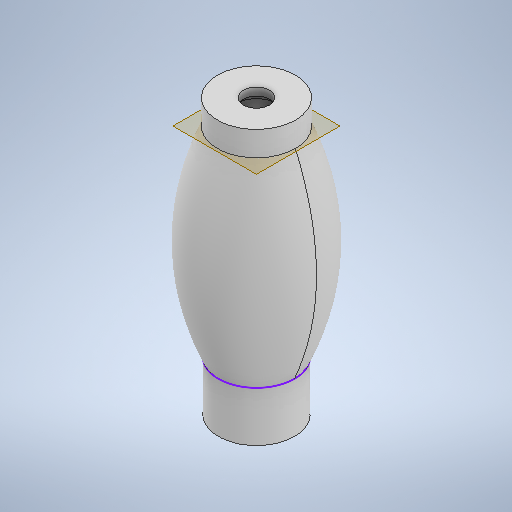
# Autodesk Inventor part: Pressure tank, 3d print. rev 001 inventor file
Saved by Autodesk Inventor 2025.2 (Build 292293000, 293)
## iProperties
Created: 2025-03-20
Part Number: Pressure tank, 3d print. rev 001 inventor file
Material: Generic
Document SubType Name: Modeling
Designer: Tobias
Density: 1 g/cm^3
Appearance: Default
Author: Tobias
## iProperties of the stored document Pressure tank, 3d print. rev 001 inventor file_3DPrint.ipt
Created: 2025-03-20
Part Number: Pressure tank, 3d print. rev 001 inventor file_3DPrint
Material: Generic
Document SubType Name: Modeling
Designer: Tobias
Density: 1 g/cm^3
Appearance: Default
Author: Tobias
Autodesk Inventor part; units mm, degrees
ref_plane "YZ Plane" through (0, 0, 0) normal (1, 0, 0) x (0, 1, 0)
ref_plane "XZ Plane" through (0, 0, 0) normal (0, 1, 0) x (-1, 0, 0)
ref_plane "XY Plane" through (0, 0, 0) normal (0, 0, 1) x (1, 0, 0)
sketch "Sketch1" plane through (0, 0, 0) normal (0, 1, 0) x (-1, 0, 0)
  circle A0 centre (0, 0) radius 15
  circle A1 centre (0, 0) radius 19
  dimension "d0" = 30
  dimension "d1" = 38
  constraints: 2 centre point, 2 coincident
  measures "d0" diameter of A0
  measures "d1" diameter of A1
extrude "Extrusion1" add sketch "Sketch1" along normal blind 25 contours A0 | A1
sketch "Sketch2" plane through (0, 25, 0) normal (0, 1, 0) x (1, 0, 0)
  circle A0 centre (0, 0) radius 19
  constraints: 1 centre point, 1 coincident
ref_plane "Work Plane1" through (0, 75, 0) normal (0, 1, 0) x (1, 0, 0)
sketch "Sketch3" plane through (0, 75, 0) normal (0, 1, 0) x (1, 0, 0)
  circle A0 centre (0, 0) radius 30
  dimension "d5" = 60
  constraints: 1 centre point, 1 coincident
  measures "d5" diameter of A0
ref_plane "Work Plane2" through (0, 125, 0) normal (0, 1, 0) x (1, 0, 0)
sketch "Sketch4" plane through (0, 125, 0) normal (0, 1, 0) x (1, 0, 0)
  point P0 (0, 0)
sketch "Sketch5" plane through (0, 125, 0) normal (0, 1, 0) x (1, 0, 0)
  circle A0 centre (0, 0) radius 19.5
  dimension "d7" = 39
  constraints: 1 centre point, 1 coincident
  measures "d7" diameter of A0
loft "Loft1" add profiles "Sketch3", "Sketch5" section 1 edges at (19, 25, 0)
sketch "Sketch7" plane through (0, 0, 0) normal (0, -1, 0) x (1, 0, 0)
  point P0 (0, 0)
  point P1 (0, 0)
  constraints: 1 coincident
hole "Hole1" at (0, 0, 0) direction (0, 1, 0) diameter 19.842 end through all clearance for "Hex Head Bolt" size "3/4" standard "Ansi Unified Screw Threads"
sketch "Sketch8" plane through (0, 125, 0) normal (0, 1, 0) x (1, 0, 0)
  circle A0 centre (0, 0) radius 19.5
  constraints: 1 centre point, 1 coincident
extrude "Extrusion2" add sketch "Sketch8" along normal blind 12.3
sketch "Sketch9" plane through (0, 137.3, 0) normal (0, 1, 0) x (1, 0, 0)
  point P0 (0, 0)
  point P1 (0, 0)
  constraints: 1 coincident
hole "Hole2" at (0, 137.3, 0) direction (0, -1, 0) diameter 13 depth 42.05 tip angle 118
sketch "Sketch10" plane through (0, 25, 0) normal (0, 1, 0) x (1, 0, 0)
  circle A0 centre (0, 0) radius 18.6
  dimension "d30" = 37.2
  constraints: 1 centre point, 1 coincident
  measures "d30" diameter of A0
sketch "Sketch11" plane through (0, 75, 0) normal (0, 1, 0) x (1, 0, 0)
  circle A0 centre (0, 0) radius 23.6
  dimension "d31" = 47.2
  constraints: 1 centre point, 1 coincident
  measures "d31" diameter of A0
sketch "Sketch12" plane through (0, 125, 0) normal (0, 1, 0) x (1, 0, 0)
  circle A0 centre (0, 0) radius 18.1
  dimension "d32" = 36.2
  constraints: 1 centre point, 1 coincident
  measures "d32" diameter of A0
loft "Loft2" cut profiles "Sketch10", "Sketch11", "Sketch12"
thread "Thread1" size "1/2" designation "1/2 - 14 NPT" standard "NPT" length 19.85
sketch "Sketch13" plane through (0, 137.3, 0) normal (0, 1, 0) x (1, 0, 0)
  circle A0 centre (0, 0) radius 10
  dimension "d41" = 20
  constraints: 1 centre point, 1 coincident
  measures "d41" diameter of A0
extrude "Extrusion3" cut sketch "Sketch13" along normal blind 8.4125 from surface at -12.3
fillet "Fillet1" radius 3.5875 1 edges at (-10, 133.4125, 0)
fillet "Fillet2" radius 8.35 1 edges at (-18.1, 125, 0)
fillet "Fillet3" radius 8.35 1 edges at (-18.6, 25, 0)
body "Solid1"
